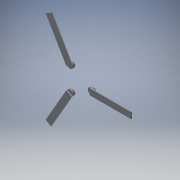
# Autodesk Inventor part: Cutting_Cable
Saved by Autodesk Inventor 2019 (Build 230136000, 136)
## iProperties
Created: 2019-03-03
Part Number: Cutting_Cable
Material: Generic
Document SubType Name: Modeling
Designer: alarr
Density: 1 g/cm^3
Appearance: Default
Author: alarr
Autodesk Inventor part; units mm, degrees
ref_plane "YZ Plane" through (0, 0, 0) normal (1, 0, 0) x (0, 1, 0)
ref_plane "XZ Plane" through (0, 0, 0) normal (0, 1, 0) x (-1, 0, 0)
sketch "Sketch1" plane through (0, 0, 0) normal (0, 0, 1) x (1, 0, 0)
  circle A0 centre (31.75, 0) radius 6.985 projected
  circle A1 centre (-15.875, -27.4963) radius 6.985 projected
  circle A2 centre (-15.875, 27.4963) radius 6.985 projected
  circle A3 centre (31.75, 0) radius 6.985
  circle A4 centre (-15.875, -27.4963) radius 6.985
  circle A5 centre (-15.875, 27.4963) radius 6.985
  point P0 (0, 0)
  constraints: 3 centre point, 3 coincident, 3 concentric
ref_plane "Work Plane1" through (-22.86, 20.5113, -5.08) normal (0, 0, 1) x (1, 0, 0)
extrude "Extrusion1" add sketch "Sketch1" against normal up to surface (5.08 mm away)
sketch "Sketch2" plane through (31.75, 0, 0) normal (0, 0, 1) x (1, 0, 0)
  circle A0 centre (-47.625, 27.4963) radius 6.985 projected
  circle A1 centre (-47.625, -27.4963) radius 6.985 projected
  circle A2 centre (0, 0) radius 6.985 projected
  line L0 (0, 6.985) -> (93.98, 6.985)
  line L1 (93.98, 6.985) -> (93.98, -6.985)
  line L2 (93.98, -6.985) -> (0, -6.985)
  line L3 (0, -6.985) -> (0, 6.985)
  point P0 (-31.75, 0)
  dimension "d2" = 93.98
  constraints: 8 end point, 3 horizontal, 2 parallel, 1 perpendicular, 1 vertical alignment, 1 other
  measures "d2" distance of L1.end L2.end
extrude "Extrusion2" add sketch "Sketch2" along normal blind 2.54 contours A2 L3 | A2 L0 L1 L2 picked at (1.4517, 1.8204)
pattern_circular "Circular Pattern1" count 3 over 360 about axis through (0, 0, -10) along (0, 0, 1) of "Extrusion2"
body "Solid1"
